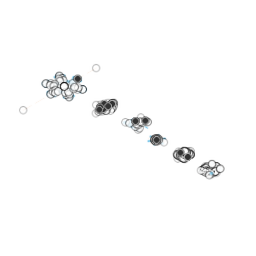
day2_sketches (Autodesk Fusion 360 design; units mm, degrees)
part number: 2026-04-13-20-48-34-590
Autodesk Fusion 360 part; units mm, degrees
(part 1 of 3)
sketch "Sketch1" plane through (0, 0, 0) normal (0, 0, 1) x (1, 0, 0)
  circle A0 centre (0, 0) radius 14
  circle A1 centre (0, 0) radius 20
  circle A2 centre (0, 0) radius 73 construction
  arc A3 (73, 0) -> (70.5126, 18.8938) centre (0, 0) ccw construction
  line L0 (0, 0) -> (73, 0) construction
  line L1 (19.3185, 5.1764) -> (34.7733, 9.3175)
  line L2 (19.3185, -5.1764) -> (34.7733, -9.3175)
  line L3 (34.7733, 9.3175) -> (73, 0)
  line L4 (34.7733, -9.3175) -> (73, 0)
  arc A4 (34.7733, -9.3175) -> (34.7733, 9.3175) centre (0, 0) ccw
  line L5 (5.1764, 19.3185) -> (9.3175, 34.7733)
  arc A5 (25.4558, 25.4558) -> (9.3175, 34.7733) centre (0, 0) ccw
  line L6 (14.1421, 14.1421) -> (25.4558, 25.4558)
  line L7 (25.4558, 25.4558) -> (36.5, 63.2199)
  line L8 (9.3175, 34.7733) -> (36.5, 63.2199)
  line L9 (-14.1421, 14.1421) -> (-25.4558, 25.4558)
  arc A6 (-9.3175, 34.7733) -> (-25.4558, 25.4558) centre (0, 0) ccw
  line L10 (-5.1764, 19.3185) -> (-9.3175, 34.7733)
  line L11 (-9.3175, 34.7733) -> (-36.5, 63.2199)
  line L12 (-25.4558, 25.4558) -> (-36.5, 63.2199)
  line L13 (-19.3185, -5.1764) -> (-34.7733, -9.3175)
  arc A7 (-34.7733, 9.3175) -> (-34.7733, -9.3175) centre (0, 0) ccw
  line L14 (-19.3185, 5.1764) -> (-34.7733, 9.3175)
  line L15 (-34.7733, 9.3175) -> (-73, 0)
  line L16 (-34.7733, -9.3175) -> (-73, 0)
  line L17 (-5.1764, -19.3185) -> (-9.3175, -34.7733)
  arc A8 (-25.4558, -25.4558) -> (-9.3175, -34.7733) centre (0, 0) ccw
  line L18 (-14.1421, -14.1421) -> (-25.4558, -25.4558)
  line L19 (-25.4558, -25.4558) -> (-36.5, -63.2199)
  line L20 (-9.3175, -34.7733) -> (-36.5, -63.2199)
  line L21 (14.1421, -14.1421) -> (25.4558, -25.4558)
  arc A9 (9.3175, -34.7733) -> (25.4558, -25.4558) centre (0, 0) ccw
  line L22 (5.1764, -19.3185) -> (9.3175, -34.7733)
  line L23 (9.3175, -34.7733) -> (36.5, -63.2199)
  line L24 (25.4558, -25.4558) -> (36.5, -63.2199)
  line L25 (300, 50) -> (350, 50) construction
  line L26 (325, 70) -> (325, 30) construction
  line L27 (300, 50) -> (300.1627, 50)
  line L28 (300.1627, 50) -> (300.1627, -30) construction
  line L29 (300.1627, -30) -> (300, -30)
  line L30 (300, -30) -> (300, 50) construction
  line L31 (260, 10) -> (370.6155, 10) construction
  arc A10 (341.6667, -42.4722) -> (308.3333, -42.4722) centre (325, -67.4166) ccw
  arc A11 (359.0765, 38.2526) -> (355.3385, 36.4191) centre (370.6155, 10) ccw
  arc A12 (300.1627, -15.0009) -> (300, -15) centre (300, -30) ccw
  arc A13 (285, -30) -> (315, -30) centre (300, -30) ccw
  arc A14 (300.1627, -20.0013) -> (300, -20) centre (300, -30) ccw
  arc A15 (290, -30) -> (310, -30) centre (300, -30) ccw
  arc A16 (340, -30) -> (360, -30) centre (350, -30) ccw
  arc A17 (335, -30) -> (365, -30) centre (350, -30) ccw
  line L32 (275, -30) -> (375, -30) construction
  arc A18 (310, -30) -> (290, -30) centre (300, -30) ccw
  arc A19 (315, -30) -> (285, -30) centre (300, -30) ccw
  arc A20 (308.3333, -17.5278) -> (341.6667, -17.5278) centre (325, 7.4166) ccw
  arc A21 (365, -30) -> (335, -30) centre (350, -30) ccw
  arc A22 (360, -30) -> (340, -30) centre (350, -30) ccw
  arc A23 (341.6667, 37.5278) -> (308.3333, 37.5278) centre (325, 12.5834) ccw
  arc A24 (308.3333, 62.4722) -> (341.6667, 62.4722) centre (325, 87.4166) ccw
  arc A25 (335, 50) -> (365, 50) centre (350, 50) ccw
  arc A26 (365, 50) -> (335, 50) centre (350, 50) ccw
  arc A27 (360, 50) -> (340, 50) centre (350, 50) ccw
  arc A28 (340, 50) -> (360, 50) centre (350, 50) ccw
  arc A29 (285, 50) -> (315, 50) centre (300, 50) ccw
  arc A30 (315, 50) -> (285, 50) centre (300, 50) ccw
  arc A31 (310, 50) -> (290, 50) centre (300, 50) ccw
  arc A32 (290, 50) -> (310, 50) centre (300, 50) ccw
  arc A33 (356.8719, 36.6667) -> (356.8719, -16.6667) centre (370.6155, 10) ccw
  arc A34 (293.1282, -16.6667) -> (293.1282, 36.6667) centre (279.3845, 10) ccw
  dimension "d7" = 360
  constraint coincident A0.centre A1.centre
  constraint concentric A1 A2
  constraint concentric A1 A4
  constraint coincident A2 A3.start
  constraint coincident A1 L2.start
  constraint coincident A1 L1.start
  constraint horizontal L25
  constraint perpendicular L25 L26
  constraint horizontal L27
  constraint vertical L28
  constraint horizontal L29
  constraint vertical L30
  constraint perpendicular L28 L31
  constraint coincident L31.end A11.centre
  constraint tangent A10 A17
  constraint tangent A10 A13
  constraint coincident A10.end A13
  constraint coincident A10.start A17
  constraint coincident L28 A12.start
  constraint coincident L30 A12.end
  constraint concentric A12 A13
  constraint coincident L28 A14.start
  constraint coincident L30 A14.end
  constraint concentric A14 A15
  constraint perpendicular L28 L32
  constraint symmetric A10.end L32 A20.start
  constraint symmetric A10.start L32 A20.end
  constraint symmetric A10 L32 A20
  constraint symmetric A13.end L32 A19.start
  constraint symmetric A17.start L32 A21.end
  constraint symmetric A13.start L32 A19.end
  constraint symmetric A13 L32 A19
  constraint symmetric A15.end L32 A18.start
  constraint symmetric A15.start L32 A18.end
  constraint symmetric A15 L32 A18
  constraint symmetric A16.end L32 A22.start
  constraint symmetric A16.start L32 A22.end
  constraint symmetric A16 L32 A22
  constraint symmetric A17.end L32 A21.start
  constraint symmetric A17 L32 A21
  constraint symmetric L31 A10.end A24.start
  constraint symmetric L31 A10.start A24.end
  constraint symmetric L31 A10 A24
  constraint symmetric L31 A13.end A29.end
  constraint symmetric L31 A17.start A25.start
  constraint symmetric L31 A13.start A29.start
  constraint symmetric L31 A13 A30
  constraint symmetric L31 A15.end A31.start
  constraint symmetric L31 A15.start A31.end
  constraint symmetric L31 A15 A31
  constraint symmetric L31 A16.end A27.start
  constraint symmetric L31 A16.start A27.end
  constraint symmetric L31 A16 A27
  constraint symmetric L31 A17.end A25.end
  constraint symmetric L31 A17 A26
  constraint symmetric L31 A18 A32
  constraint symmetric L31 A19 A29
  constraint symmetric L31 A20.end A23.start
  constraint symmetric L31 A20.start A23.end
  constraint symmetric L31 A20 A23
  constraint symmetric L31 A21 A25
  constraint symmetric L31 A22 A28
  constraint tangent A25 A33
  constraint coincident A21 A33.end
  constraint coincident A25 A33.start
  constraint coincident L31 A34.centre
  constraint tangent A29 A34
  constraint coincident A29 A34.end
  constraint coincident A19 A34.start
sketch "Sketch2" plane through (0, 0, 0) normal (0, 0, 1) x (1, 0, 0)
  line L0 (-379.9986, -15) -> (-214.9986, -15)
  line L1 (-214.9986, -15) -> (-214.9986, -5.344)
  line L2 (-219.9986, -0.344) -> (-226.0015, -0.344)
  line L3 (-379.9986, -5.344) -> (-379.9986, -15)
  arc A0 (-214.9986, -5.344) -> (-219.9986, -0.344) centre (-219.9986, -5.344) ccw
  arc A1 (-374.9986, -0.344) -> (-379.9986, -5.344) centre (-374.9986, -5.344) ccw
  circle A2 centre (-326, 69) radius 16
  circle A3 centre (-326, 69) radius 35
  line L4 (-326, 69) -> (-325.9604, 133.975) construction
  line L5 (-325.9604, 133.975) -> (-271.0015, 133.9415) construction
  circle A4 centre (-271.0015, 133.9415) radius 12
  circle A5 centre (-271.0015, 133.9415) radius 25
  line L6 (-246.0015, 133.9415) -> (-246.0015, 132)
  line L7 (-271.0015, 133.9415) -> (-241, 133.9415) construction
  line L8 (-246.0015, 133.9415) -> (-246.0015, 19.656)
  arc A6 (-246.0015, 19.656) -> (-226.0015, -0.344) centre (-226.0015, 19.656) ccw
  arc A7 (-328.4008, 103.9176) -> (-295.9182, 135.9805) centre (-330.8016, 138.8351) ccw
  line L9 (-261.0635, 111.0016) -> (-261.0635, 92.814)
  line L10 (-326, 69) -> (-180, 68.9111) construction
  line L11 (-180, 68.9111) -> (-206.1133, 68.927)
  line L12 (-290.1965, 84.814) -> (-269.0635, 84.814)
  line L13 (-290.2427, 53.1529) -> (-269.8408, 53.2148)
  line L14 (-261.777, 8.7586) -> (-261.8166, 45.2235)
  line L15 (-374.9986, -0.344) -> (-225, -0.344)
  arc A8 (-360.0045, 60.712) -> (-268.3878, 0.8714) centre (-282.2799, 79.656) ccw
  arc A9 (-268.3878, 0.8714) -> (-261.777, 8.7586) centre (-269.777, 8.7499) ccw
  arc A10 (-261.8166, 45.2235) -> (-269.8408, 53.2148) centre (-269.8166, 45.2148) ccw
  arc A11 (-269.0635, 84.814) -> (-261.0635, 92.814) centre (-269.0635, 92.814) ccw
  arc A12 (-290.2427, 53.1529) -> (-296.8755, 49.5896) centre (-290.2184, 45.153) ccw
  arc A13 (-296.8576, 88.3835) -> (-290.1965, 84.814) centre (-290.1965, 92.814) ccw
  arc A14 (-338.8484, -0.344) -> (-332.563, 17.4338) centre (-338.8484, 9.656) ccw
  line L16 (-650, 60) -> (-698, 60)
  circle A15 centre (-698, 60) radius 7.5
  line L17 (-650, 60) -> (-650, 108) construction
  line L18 (-664, 108) -> (-664, 94)
  line L19 (-698, 74) -> (-684, 74)
  arc A16 (-684, 74) -> (-664, 94) centre (-684, 94) ccw
  arc A17 (-697.4782, 13.3614) -> (-703.1993, 47.0013) centre (-710.6269, 28.4316) ccw
  arc A18 (-703.9799, -1.4739) -> (-650, -54) centre (-650, 0) ccw
  arc A19 (-698, 74) -> (-703.1993, 47.0013) centre (-698, 60) ccw
  arc A20 (-650, 122) -> (-664, 108) centre (-650, 108) ccw
  arc A21 (-650, 115.5) -> (-650, 100.5) centre (-650, 108) ccw
  line L20 (-650, 130) -> (-650, -90) construction
  line L21 (-650, 0) -> (-736.423, 0) construction
  line L22 (-650, 0) -> (-677, -46.7654) construction
  arc A22 (-676, 0) -> (-663, -22.5167) centre (-650, 0) ccw
  arc A23 (-694, 0) -> (-672, -38.1051) centre (-650, 0) ccw
  arc A24 (-676, 0) -> (-694, 0) centre (-685, 0) ccw
  arc A25 (-672, -38.1051) -> (-663, -22.5167) centre (-667.5, -30.3109) ccw
  line L23 (-660, 60) -> (-660, 20)
  arc A26 (-662, 16) -> (-660, 20) centre (-665, 20) ccw
  arc A27 (-650, 70) -> (-650, 50) centre (-650, 60) ccw
  arc A28 (-662, 16) -> (-650, -20) centre (-650, 0) ccw
  arc A29 (-650, 35) -> (-650, -35) centre (-650, 0) ccw construction
  arc A30 (-650, 100.5) -> (-650, 115.5) centre (-650, 108) ccw
  line L24 (-636, 108) -> (-636, 94)
  arc A31 (-636, 108) -> (-650, 122) centre (-650, 108) ccw
  arc A32 (-636, 94) -> (-616, 74) centre (-616, 94) ccw
  line L25 (-602, 74) -> (-616, 74)
  arc A33 (-596.8007, 47.0013) -> (-602, 74) centre (-602, 60) ccw
  circle A34 centre (-602, 60) radius 7.5
  arc A35 (-650, 50) -> (-650, 70) centre (-650, 60) ccw
  line L26 (-640, 60) -> (-640, 20)
  arc A36 (-596.8007, 47.0013) -> (-602.5218, 13.3614) centre (-589.3731, 28.4316) ccw
  arc A37 (-650, -54) -> (-596.0201, -1.4739) centre (-650, 0) ccw
  arc A38 (-628, -38.1051) -> (-606, 0) centre (-650, 0) ccw
  arc A39 (-637, -22.5167) -> (-624, 0) centre (-650, 0) ccw
  arc A40 (-637, -22.5167) -> (-628, -38.1051) centre (-632.5, -30.3109) ccw
  arc A41 (-606, 0) -> (-624, 0) centre (-615, 0) ccw
  arc A42 (-650, -20) -> (-638, 16) centre (-650, 0) ccw
  arc A43 (-640, 20) -> (-638, 16) centre (-635, 20) ccw
  arc A44 (-596.0201, -1.4739) -> (-602.5218, 13.3614) centre (-615.013, -0.9553) ccw
  arc A45 (-697.4782, 13.3614) -> (-703.9799, -1.4739) centre (-684.987, -0.9553) ccw
  circle A46 centre (-1125, 0) radius 75
  circle A47 centre (-1125, 0) radius 90
  line L27 (-1124.6288, 388.2293) -> (-1124.6288, -500) construction
  line L28 (-1139.6288, 121.5732) -> (-1139.6288, 88.8031)
  line L29 (-1109.6288, 121.5732) -> (-1109.6288, 88.8031)
  circle A48 centre (-1124.6288, 163.9996) radius 30
  arc A49 (-1169.2171, 157.9267) -> (-1080.0684, 157.7249) centre (-1124.6288, 163.9996) ccw
  arc A50 (-1080.0684, 157.7249) -> (-1169.2171, 157.9267) centre (-1125, 0) ccw
  circle A51 centre (-1266.8422, 82.3213) radius 30
  arc A52 (-1239.128, 117.7744) -> (-1283.8771, 40.6702) centre (-1125, 0) ccw
  arc A53 (-1283.8771, 40.6702) -> (-1239.128, 117.7744) centre (-1266.8422, 82.3213) ccw
  line L30 (-1222.5998, 74.0985) -> (-1194.2202, 57.7134)
  line L31 (-1237.5998, 48.1177) -> (-1209.2202, 31.7327)
  circle A54 centre (-1267.2134, -81.6783) radius 30
  arc A55 (-1284.0596, -39.9505) -> (-1239.66, -117.2565) centre (-1125, 0) ccw
  arc A56 (-1239.66, -117.2565) -> (-1284.0596, -39.9505) centre (-1267.2134, -81.6783) ccw
  line L32 (-1237.9711, -47.4747) -> (-1209.5914, -31.0897)
  line L33 (-1222.9711, -73.4555) -> (-1194.5914, -57.0705)
  circle A57 centre (-1125.3712, -163.9996) radius 30
  arc A58 (-1169.9316, -157.7249) -> (-1080.7829, -157.9267) centre (-1125, 0) ccw
  arc A59 (-1080.7829, -157.9267) -> (-1169.9316, -157.7249) centre (-1125.3712, -163.9996) ccw
  line L34 (-1140.3712, -121.5732) -> (-1140.3712, -88.8031)
  line L35 (-1110.3712, -121.5732) -> (-1110.3712, -88.8031)
  circle A60 centre (-983.1578, -82.3213) radius 30
  arc A61 (-1010.872, -117.7744) -> (-966.1229, -40.6702) centre (-1125, 0) ccw
  arc A62 (-966.1229, -40.6702) -> (-1010.872, -117.7744) centre (-983.1578, -82.3213) ccw
  line L36 (-1027.4002, -74.0985) -> (-1055.7798, -57.7134)
  line L37 (-1012.4002, -48.1177) -> (-1040.7798, -31.7327)
  circle A63 centre (-982.7866, 81.6783) radius 30
  arc A64 (-965.9404, 39.9505) -> (-1010.34, 117.2565) centre (-1125, 0) ccw
  arc A65 (-1010.34, 117.2565) -> (-965.9404, 39.9505) centre (-982.7866, 81.6783) ccw
  line L38 (-1012.0289, 47.4747) -> (-1040.4086, 31.0897)
  line L39 (-1027.0289, 73.4555) -> (-1055.4086, 57.0705)
  line L40 (597.5, -18) -> (608.5, -18)
  line L41 (609, -17.5) -> (609, -14.5)
  line L42 (608.5, -14) -> (597.5, -14)
  line L43 (597, -14.5) -> (597, -17.5)
  line L44 (597.5, -13) -> (604.5, -13)
  line L45 (605, -12.5) -> (605, -9.5)
  line L46 (604.5, -9) -> (597.5, -9)
  line L47 (597, -9.5) -> (597, -12.5)
  line L48 (597.5, -8) -> (602.5, -8)
  line L49 (603, -7.5) -> (603, -4.5)
  line L50 (602.5, -4) -> (597.5, -4)
  line L51 (597, -4.5) -> (597, -7.5)
  line L52 (604.5, -4) -> (607.5, -4)
  line L53 (608, -4.5) -> (608, -7.5)
  line L54 (607.5, -8) -> (604.5, -8)
  line L55 (604, -7.5) -> (604, -4.5)
  line L56 (612.5, -8) -> (609.5, -8)
  line L57 (609, -7.5) -> (609, -4.5)
  line L58 (613, -4.5) -> (613, -7.5)
  line L59 (609.5, -4) -> (612.5, -4)
  line L60 (617.5, -8) -> (614.5, -8)
  line L61 (614, -7.5) -> (614, -4.5)
  line L62 (618, -4.5) -> (618, -7.5)
  line L63 (614.5, -4) -> (617.5, -4)
  line L64 (622.5, -8) -> (619.5, -8)
  line L65 (619, -7.5) -> (619, -4.5)
  line L66 (623, -4.5) -> (623, -7.5)
  line L67 (619.5, -4) -> (622.5, -4)
  line L68 (627.5, -8) -> (624.5, -8)
  line L69 (624, -7.5) -> (624, -4.5)
  line L70 (628, -4.5) -> (628, -7.5)
  line L71 (624.5, -4) -> (627.5, -4)
  line L72 (632.5, -8) -> (629.5, -8)
  line L73 (629, -7.5) -> (629, -4.5)
  line L74 (633, -4.5) -> (633, -7.5)
  line L75 (629.5, -4) -> (632.5, -4)
  line L76 (637.5, -8) -> (634.5, -8)
  line L77 (634, -7.5) -> (634, -4.5)
  line L78 (638, -4.5) -> (638, -7.5)
  line L79 (634.5, -4) -> (637.5, -4)
  line L80 (642.5, -8) -> (639.5, -8)
  line L81 (639, -7.5) -> (639, -4.5)
  line L82 (643, -4.5) -> (643, -7.5)
  line L83 (639.5, -4) -> (642.5, -4)
  line L84 (647.5, -8) -> (644.5, -8)
  line L85 (644, -7.5) -> (644, -4.5)
  line L86 (648, -4.5) -> (648, -7.5)
  line L87 (644.5, -4) -> (647.5, -4)
  line L88 (652.5, -8) -> (649.5, -8)
  line L89 (649, -7.5) -> (649, -4.5)
  line L90 (653, -4.5) -> (653, -7.5)
  line L91 (649.5, -4) -> (652.5, -4)
  line L92 (657.5, -8) -> (654.5, -8)
  line L93 (654, -7.5) -> (654, -4.5)
  line L94 (658, -4.5) -> (658, -7.5)
  line L95 (654.5, -4) -> (657.5, -4)
  line L96 (662.5, -8) -> (659.5, -8)
  line L97 (659, -7.5) -> (659, -4.5)
  line L98 (663, -4.5) -> (663, -7.5)
  line L99 (659.5, -4) -> (662.5, -4)
  line L100 (667.5, -8) -> (664.5, -8)
  line L101 (664, -7.5) -> (664, -4.5)
  line L102 (668, -4.5) -> (668, -7.5)
  line L103 (664.5, -4) -> (667.5, -4)
  line L104 (606.5, -9) -> (609.5, -9)
  line L105 (610, -9.5) -> (610, -12.5)
  line L106 (609.5, -13) -> (606.5, -13)
  line L107 (606, -12.5) -> (606, -9.5)
  line L108 (614.5, -13) -> (611.5, -13)
  line L109 (611, -12.5) -> (611, -9.5)
  line L110 (611.5, -9) -> (614.5, -9)
  line L111 (615, -9.5) -> (615, -12.5)
  line L112 (619.5, -13) -> (616.5, -13)
  line L113 (616, -12.5) -> (616, -9.5)
  line L114 (616.5, -9) -> (619.5, -9)
  line L115 (620, -9.5) -> (620, -12.5)
  line L116 (624.5, -13) -> (621.5, -13)
  line L117 (621, -12.5) -> (621, -9.5)
  line L118 (621.5, -9) -> (625, -9)
  line L119 (625, -9) -> (625, -12.5)
  line L120 (629.5, -13) -> (626.5, -13)
  line L121 (626, -12.5) -> (626, -9.5)
  line L122 (626.5, -9) -> (629.5, -9)
  line L123 (630, -9.5) -> (630, -12.5)
  line L124 (634.5, -13) -> (631.5, -13)
  line L125 (631, -12.5) -> (631, -9.5)
  line L126 (631.5, -9) -> (634.5, -9)
  line L127 (635, -9.5) -> (635, -12.5)
  line L128 (639.5, -13) -> (636.5, -13)
  line L129 (636, -12.5) -> (636, -9.5)
  line L130 (636.5, -9) -> (639.5, -9)
  line L131 (640, -9.5) -> (640, -12.5)
  line L132 (644.5, -13) -> (641.5, -13)
  line L133 (641, -12.5) -> (641, -9.5)
  line L134 (641.5, -9) -> (644.5, -9)
  line L135 (645, -9.5) -> (645, -12.5)
  line L136 (649.5, -13) -> (646.5, -13)
  line L137 (646, -12.5) -> (646, -9.5)
  line L138 (646.5, -9) -> (649.5, -9)
  line L139 (650, -9.5) -> (650, -12.5)
  line L140 (654.5, -13) -> (651.5, -13)
  line L141 (651, -12.5) -> (651, -9.5)
  line L142 (651.5, -9) -> (654.5, -9)
  line L143 (655, -9.5) -> (655, -12.5)
  line L144 (659.5, -13) -> (656.5, -13)
  line L145 (656, -12.5) -> (656, -9.5)
  line L146 (656.5, -9) -> (659.5, -9)
  line L147 (660, -9.5) -> (660, -12.5)
  line L148 (661.5, -9) -> (667.5, -9)
  line L149 (668, -9.5) -> (668, -12.5)
  line L150 (667.5, -13) -> (661.5, -13)
  line L151 (661, -12.5) -> (661, -9.5)
  line L152 (610.5, -14) -> (613.5, -14)
  line L153 (614, -14.5) -> (614, -17.5)
  line L154 (613.5, -18) -> (610.5, -18)
  line L155 (610, -17.5) -> (610, -14.5)
  line L156 (618.5, -18) -> (615.5, -18)
  line L157 (615, -17.5) -> (615, -14.5)
  line L158 (615.5, -14) -> (618.5, -14)
  line L159 (619, -14.5) -> (619, -17.5)
  line L160 (623.5, -18) -> (620.5, -18)
  line L161 (620, -17.5) -> (620, -14.5)
  line L162 (620.5, -14) -> (623.5, -14)
  line L163 (624, -14.5) -> (624, -17.5)
  line L164 (628.5, -18) -> (625.5, -18)
  line L165 (625, -17.5) -> (625, -14.5)
  line L166 (625.5, -14) -> (628.5, -14)
  line L167 (629, -14.5) -> (629, -17.5)
  line L168 (633.5, -18) -> (630.5, -18)
  line L169 (630, -17.5) -> (630, -14)
  line L170 (630, -14) -> (633.5, -14)
  line L171 (634, -14.5) -> (634, -17.5)
  line L172 (638.5, -18) -> (635.5, -18)
  line L173 (635, -17.5) -> (635, -14.5)
  line L174 (635.5, -14) -> (638.5, -14)
  line L175 (639, -14.5) -> (639, -17.5)
  line L176 (643.5, -18) -> (640.5, -18)
  line L177 (640, -17.5) -> (640, -14.5)
  line L178 (640.5, -14) -> (643.5, -14)
  line L179 (644, -14.5) -> (644, -17.5)
  line L180 (648.5, -18) -> (645.5, -18)
  line L181 (645, -17.5) -> (645, -14.5)
  line L182 (645.5, -14) -> (648.5, -14)
  line L183 (649, -14.5) -> (649, -17.5)
  line L184 (653.5, -18) -> (650.5, -18)
  line L185 (650, -17.5) -> (650, -14.5)
  line L186 (650.5, -14) -> (653.5, -14)
  line L187 (654, -14.5) -> (654, -17.5)
  line L188 (658.5, -18) -> (655.5, -18)
  line L189 (655, -17.5) -> (655, -14.5)
  line L190 (655.5, -14) -> (658.5, -14)
  line L191 (659, -14.5) -> (659, -17.5)
  line L192 (660.5, -14) -> (667.5, -14)
  line L193 (668, -14.5) -> (668, -17.5)
  line L194 (667.5, -18) -> (660.5, -18)
  line L195 (660, -17.5) -> (660, -14.5)
  line L196 (597.5, -3) -> (599.5, -3)
  line L197 (600, -2.5) -> (600, 0.5)
  line L198 (599.5, 1) -> (597.5, 1)
  line L199 (597, 0.5) -> (597, -2.5)
  line L200 (601.5, 1) -> (604.5, 1)
  line L201 (605, 0.5) -> (605, -2.5)
  line L202 (604.5, -3) -> (601.5, -3)
  line L203 (601, -2.5) -> (601, 0.5)
  line L204 (609.5, -3) -> (606.5, -3)
  line L205 (606, -2.5) -> (606, 0.5)
  line L206 (606.5, 1) -> (609.5, 1)
  line L207 (610, 0.5) -> (610, -2.5)
  line L208 (614.5, -3) -> (611.5, -3)
  line L209 (611, -2.5) -> (611, 0.5)
  line L210 (611.5, 1) -> (614.5, 1)
  line L211 (615, 0.5) -> (615, -2.5)
  line L212 (619.5, -3) -> (616.5, -3)
  line L213 (616, -2.5) -> (616, 0.5)
  line L214 (616.5, 1) -> (619.5, 1)
  line L215 (620, 0.5) -> (620, -2.5)
  line L216 (624.5, -3) -> (621.5, -3)
  line L217 (621, -2.5) -> (621, 0.5)
  line L218 (621.5, 1) -> (624.5, 1)
  line L219 (625, 0.5) -> (625, -2.5)
  line L220 (629.5, -3) -> (626.5, -3)
  line L221 (626, -2.5) -> (626, 0.5)
  line L222 (626.5, 1) -> (629.5, 1)
  line L223 (630, 0.5) -> (630, -2.5)
  line L224 (634.5, -3) -> (631.5, -3)
  line L225 (631, -2.5) -> (631, 0.5)
  line L226 (631.5, 1) -> (634.5, 1)
  line L227 (635, 0.5) -> (635, -2.5)
  line L228 (639.5, -3) -> (636.5, -3)
  line L229 (636, -2.5) -> (636, 0.5)
  line L230 (636.5, 1) -> (639.5, 1)
  line L231 (640, 0.5) -> (640, -2.5)
  line L232 (644.5, -3) -> (641.5, -3)
  line L233 (641, -2.5) -> (641, 0.5)
  line L234 (641.5, 1) -> (644.5, 1)
  line L235 (645, 0.5) -> (645, -2.5)
  line L236 (649.5, -3) -> (646.5, -3)
  line L237 (646, -2.5) -> (646, 0.5)
  line L238 (646.5, 1) -> (649.5, 1)
  line L239 (650, 0.5) -> (650, -2.5)
  line L240 (654.5, -3) -> (651.5, -3)
  line L241 (651, -2.5) -> (651, 0.5)
  line L242 (651.5, 1) -> (654.5, 1)
  line L243 (655, 0.5) -> (655, -2.5)
  line L244 (659.5, -3) -> (656.5, -3)
  line L245 (656, -2.5) -> (656, 0.5)
  line L246 (656.5, 1) -> (659.5, 1)
  line L247 (660, 0.5) -> (660, -2.5)
  line L248 (661.5, -3) -> (667.5, -3)
  line L249 (668, -2.5) -> (668, 0.5)
  line L250 (667.5, 1) -> (661.5, 1)
  line L251 (661, 0.5) -> (661, -2.5)
  line L252 (599.5007, 2) -> (602.5007, 2)
  line L253 (603.0007, 2.5) -> (603.0007, 4.5)
  line L254 (602.5007, 5) -> (599.5007, 5)
  line L255 (599.0007, 4.5) -> (599.0007, 2.5)
  line L256 (604.5007, 2) -> (607.5007, 2)
  line L257 (608.0007, 2.5) -> (608.0007, 4.5)
  line L258 (604.0007, 4.5) -> (604.0007, 2.5)
  line L259 (607.5007, 5) -> (604.5007, 5)
  line L260 (609.5007, 2) -> (612.5007, 2)
  line L261 (613.0007, 2.5) -> (613.0007, 4.5)
  line L262 (609.0007, 4.5) -> (609.0007, 2.5)
  line L263 (612.5007, 5) -> (609.5007, 5)
  line L264 (614.5007, 2) -> (617.5007, 2)
  line L265 (618.0007, 2.5) -> (618.0007, 4.5)
  line L266 (614.0007, 4.5) -> (614.0007, 2.5)
  line L267 (617.5007, 5) -> (614.5007, 5)
  line L268 (619.5007, 2) -> (622.5007, 2)
  line L269 (623.0007, 2.5) -> (623.0007, 4.5)
  line L270 (619.0007, 4.5) -> (619.0007, 2.5)
  line L271 (622.5007, 5) -> (619.5007, 5)
  line L272 (624.5007, 2) -> (627.5007, 2)
  line L273 (628.0007, 2.5) -> (628.0007, 4.5)
  line L274 (624.0007, 4.5) -> (624.0007, 2.5)
  line L275 (627.5007, 5) -> (624.5007, 5)
  line L276 (629.5007, 2) -> (632.5007, 2)
  line L277 (633.0007, 2.5) -> (633.0007, 4.5)
  line L278 (629.0007, 4.5) -> (629.0007, 2.5)
  line L279 (632.5007, 5) -> (629.5007, 5)
  line L280 (634.5007, 2) -> (637.5007, 2)
  line L281 (638.0007, 2.5) -> (638.0007, 4.5)
  line L282 (634.0007, 4.5) -> (634.0007, 2.5)
  line L283 (637.5007, 5) -> (634.5007, 5)
  line L284 (639.5007, 2) -> (642.5007, 2)
  line L285 (643.0007, 2.5) -> (643.0007, 4.5)
  line L286 (639.0007, 4.5) -> (639.0007, 2.5)
  line L287 (642.5007, 5) -> (639.5007, 5)
  line L288 (644.5007, 2) -> (647.5007, 2)
  line L289 (648.0007, 2.5) -> (648.0007, 4.5)
  line L290 (644.0007, 4.5) -> (644.0007, 2.5)
  line L291 (647.5007, 5) -> (644.5007, 5)
  line L292 (649.5007, 2) -> (652.5007, 2)
  line L293 (653.0007, 2.5) -> (653.0007, 4.5)
  line L294 (649.0007, 4.5) -> (649.0007, 2.5)
  line L295 (652.5007, 5) -> (649.5007, 5)
  line L296 (654.5007, 2) -> (657.5007, 2)
  line L297 (658.0007, 2.5) -> (658.0007, 4.5)
  line L298 (654.0007, 4.5) -> (654.0007, 2.5)
  line L299 (657.5007, 5) -> (654.5007, 5)
  line L300 (659.5007, 2) -> (662.5007, 2)
  line L301 (663.0007, 2.5) -> (663.0007, 4.5)
  line L302 (659.0007, 4.5) -> (659.0007, 2.5)
  line L303 (662.5007, 5) -> (659.5007, 5)
  line L304 (664.5007, 2) -> (667.5007, 2)
  line L305 (668.0007, 2.5) -> (668.0007, 4.5)
  line L306 (664.0007, 4.5) -> (664.0007, 2.5)
  line L307 (667.5007, 5) -> (664.5007, 5)
  line L308 (669.5007, 2) -> (672.5007, 2)
  line L309 (673.0007, 2.5) -> (673.0007, 4.5)
  line L310 (669.0007, 4.5) -> (669.0007, 2.5)
  line L311 (672.5007, 5) -> (669.5007, 5)
  line L312 (674.5007, 2) -> (677.5007, 2)
  line L313 (678.0007, 2.5) -> (678.0007, 4.5)
  line L314 (674.0007, 4.5) -> (674.0007, 2.5)
  line L315 (677.5007, 5) -> (674.5007, 5)
  line L316 (679.5007, 2) -> (682.5007, 2)
  line L317 (683.0007, 2.5) -> (683.0007, 4.5)
  line L318 (679.0007, 4.5) -> (679.0007, 2.5)
  line L319 (682.5007, 5) -> (679.5007, 5)
  line L320 (684.5007, 2) -> (687.5007, 2)
  line L321 (688.0007, 2.5) -> (688.0007, 4.5)
  line L322 (684.0007, 4.5) -> (684.0007, 2.5)
  line L323 (687.5007, 5) -> (684.5007, 5)
  line L324 (669.5, 1) -> (672.5, 1)
  line L325 (673, 0.5) -> (673, -2.5)
  line L326 (672.5, -3) -> (669.5, -3)
  line L327 (669, -2.5) -> (669, 0.5)
  line L328 (674.5, 1) -> (677.5, 1)
  line L329 (678, 0.5) -> (678, -2.5)
  line L330 (677.5, -3) -> (674.5, -3)
  line L331 (674, -2.5) -> (674, 0.5)
  line L332 (679.5, 1) -> (682.5, 1)
  line L333 (683, 0.5) -> (683, -2.5)
  line L334 (682.5, -3) -> (679.5, -3)
  line L335 (679, -2.5) -> (679, 0.5)
  line L336 (684.5, 1) -> (687.5, 1)
  line L337 (688, 0.5) -> (688, -2.5)
  line L338 (687.5, -3) -> (684.5, -3)
  line L339 (684, -2.5) -> (684, 0.5)
  line L340 (669.5, -4) -> (672.5, -4)
  line L341 (673, -4.5) -> (673, -7.5)
  line L342 (672.5, -8) -> (669.5, -8)
  line L343 (669, -7.5) -> (669, -4.5)
  line L344 (677.5, -8) -> (674.5, -8)
  line L345 (674, -7.5) -> (674, -4.5)
  line L346 (678, -4.5) -> (678, -7.5)
  line L347 (674.5, -4) -> (677.5, -4)
  line L348 (682.5, -8) -> (679.5, -8)
  line L349 (679, -7.5) -> (679, -4.5)
  line L350 (683, -4.5) -> (683, -7.5)
  line L351 (679.5, -4) -> (682.5, -4)
  line L352 (684.5, -4) -> (687.5, -4)
  line L353 (672.5, -13) -> (669.5, -13)
  line L354 (669, -12.5) -> (669, -9.5)
  line L355 (673, -9.5) -> (673, -12.5)
  line L356 (669.5, -9) -> (672.5, -9)
  line L357 (677.5, -13) -> (674.5, -13)
  line L358 (674, -12.5) -> (674, -9.5)
  line L359 (678, -9.5) -> (678, -12.5)
  line L360 (674.5, -9) -> (677.5, -9)
  line L361 (683, -13) -> (679.5, -13)
  line L362 (679, -12.5) -> (679, -9.5)
  line L363 (683, -9.5) -> (683, -13)
  line L364 (679.5, -9) -> (682.5, -9)
  line L365 (687.5, -13) -> (684.5, -13)
  line L366 (684, -12.5) -> (684, -4.5)
  line L367 (688, -4.5) -> (688, -12.5)
  line L368 (672.5, -18) -> (669.5, -18)
  line L369 (669, -17.5) -> (669, -14.5)
  line L370 (673, -14.5) -> (673, -17.5)
  line L371 (669.5, -14) -> (672.5, -14)
  line L372 (677.5, -18) -> (674.5, -18)
  line L373 (674, -17.5) -> (674, -14.5)
  line L374 (678, -14.5) -> (678, -17.5)
  line L375 (674.5, -14) -> (677.5, -14)
  line L376 (682.5, -18) -> (679.5, -18)
  line L377 (679, -17.5) -> (679, -14.5)
  line L378 (683, -14.5) -> (683, -17.5)
  line L379 (679.5, -14) -> (682.5, -14)
  line L380 (677.5, -23) -> (669.5, -23)
  line L381 (669, -22.5) -> (669, -19.5)
  line L382 (678, -19.5) -> (678, -22.5)
  line L383 (669.5, -19) -> (677.5, -19)
  line L384 (682.5, -23) -> (679.5, -23)
  line L385 (679, -22.5) -> (679, -19.5)
  line L386 (683, -19.5) -> (683, -22.5)
  line L387 (679.5, -19) -> (682.5, -19)
  line L388 (684.5, -14) -> (687.5, -14)
  line L389 (688, -14.5) -> (688, -22.5)
  line L390 (687.5, -23) -> (684.5, -23)
  line L391 (684, -22.5) -> (684, -14.5)
  line L392 (597.5, -19) -> (600.5, -19)
  line L393 (601, -19.5) -> (601, -22.5)
  line L394 (600.5, -23) -> (597.5, -23)
  line L395 (597, -22.5) -> (597, -19.5)
  line L396 (602.5, -19) -> (605.5, -19)
  line L397 (606, -19.5) -> (606, -22.5)
  line L398 (605.5, -23) -> (602.5, -23)
  line L399 (602, -22.5) -> (602, -19.5)
  line L400 (607.5, -19) -> (610.5, -19)
  line L401 (611, -19.5) -> (611, -22.5)
  line L402 (610.5, -23) -> (607.5, -23)
  line L403 (607, -22.5) -> (607, -19.5)
  line L404 (612.5, -19) -> (615.5, -19)
  line L405 (616, -19.5) -> (616, -22.5)
  line L406 (615.5, -23) -> (612.5, -23)
  line L407 (612, -22.5) -> (612, -19.5)
  line L408 (667.5, -19) -> (664.5, -19)
  line L409 (664, -19.5) -> (664, -22.5)
  line L410 (664.5, -23) -> (667.5, -23)
  line L411 (668, -22.5) -> (668, -19.5)
  line L412 (662.5, -19) -> (659.5138, -19)
  line L413 (659.0138, -19.5) -> (659.0138, -20.202)
  line L414 (659.5138, -20.702) -> (662.5, -20.702)
  line L415 (663, -20.202) -> (663, -19.5)
  line L416 (659.5138, -21.1515) -> (662.5, -21.1515)
  line L417 (663, -21.6515) -> (663, -22.5)
  line L418 (662.5, -23) -> (659.5138, -23)
  line L419 (659.0138, -22.5) -> (659.0138, -21.6515)
  line L420 (657.5, -19) -> (654.5, -19)
  line L421 (654, -19.5) -> (654, -22.5)
  line L422 (654.5, -23) -> (657.5, -23)
  line L423 (658, -22.5) -> (658, -19.5)
  line L424 (652.5, -19) -> (649.5, -19)
  line L425 (649, -19.5) -> (649, -22.5)
  line L426 (649.5, -23) -> (652.5, -23)
  line L427 (653, -22.5) -> (653, -19.5)
  line L428 (647.5, -19) -> (644.5, -19)
  line L429 (644, -19.5) -> (644, -22.5)
  line L430 (644.5, -23) -> (647.5, -23)
  line L431 (648, -22.5) -> (648, -19.5)
  line L432 (617.5, -19) -> (642.5, -19)
  line L433 (643, -19.5) -> (643, -22.5)
  line L434 (642.5, -23) -> (617.5, -23)
  line L435 (617, -22.5) -> (617, -19.5)
  line L436 (616.5, -25) -> (641, -25)
  line L437 (643, -27) -> (643, -45)
  line L438 (641, -47) -> (617, -47)
  line L439 (615, -45) -> (615, -26.5)
  line L440 (592, 10) -> (693, 10)
  line L441 (695, 8) -> (695, -53)
  line L442 (693, -55) -> (592, -55)
  line L443 (590, -53) -> (590, 8)
  line L444 (580, 15) -> (712.1237, 15) construction
  line L445 (693, 85) -> (592, 85)
  line L446 (590, 83) -> (590, 22)
  line L447 (695, 22) -> (695, 83)
  line L448 (592, 20) -> (693, 20)
  line L449 (594, 82) -> (691, 82)
  line L450 (693, 80) -> (693, 26)
  line L451 (691, 24) -> (594, 24)
  line L452 (592, 26) -> (592, 80)
  circle A66 centre (640.4399, 83.4266) radius 1.0913
  circle A67 centre (643.5479, 83.4266) radius 0.379
  circle A68 centre (645.4808, 83.4266) radius 0.379
  line L453 (600, 2.5387) -> (602.3984, 2.5387) construction
  line L454 (602.3984, 2.5387) -> (602.3984, 4) construction
  line L455 (602.3984, 4) -> (600, 4) construction
  line L456 (600, 4) -> (600, 2.5387) construction
  line L457 (605.1445, 2.6511) -> (607.8339, 2.6511) construction
  line L458 (607.8339, 2.6511) -> (607.8339, 4.0538) construction
  line L459 (607.8339, 4.0538) -> (605.1445, 4.0538) construction
  line L460 (605.1445, 4.0538) -> (605.1445, 2.6511) construction
  line L461 (610.1729, 2.7128) -> (612.2746, 2.7122) construction
  line L462 (612.2746, 2.7122) -> (612.275, 4.1069) construction
  line L463 (612.275, 4.1069) -> (610.1732, 4.1075) construction
  line L464 (610.1732, 4.1075) -> (610.1729, 2.7128) construction
  line L465 (615, 3) -> (617, 3) construction
  line L466 (617, 3) -> (617, 4) construction
  line L467 (617, 4) -> (615, 4) construction
  line L468 (615, 4) -> (615, 3) construction
  line L469 (620, 3) -> (622, 3) construction
  line L470 (622, 3) -> (622, 4) construction
  line L471 (622, 4) -> (620, 4) construction
  line L472 (620, 4) -> (620, 3) construction
  line L473 (624.8021, 2.7475) -> (627.2182, 2.7475) construction
  line L474 (627.2182, 2.7475) -> (627.2182, 4.2315) construction
  line L475 (627.2182, 4.2315) -> (624.8021, 4.2315) construction
  line L476 (624.8021, 4.2315) -> (624.8021, 2.7475) construction
  line L477 (629.7295, 2.6714) -> (632.3739, 2.6714) construction
  line L478 (632.3739, 2.6714) -> (632.3739, 4.2315) construction
  line L479 (632.3739, 4.2315) -> (629.7295, 4.2315) construction
  line L480 (629.7295, 4.2315) -> (629.7295, 2.6714) construction
  line L481 (634.8662, 2.7666) -> (637.3394, 2.7666) construction
  line L482 (637.3394, 2.7666) -> (637.3394, 4.2124) construction
  line L483 (637.3394, 4.2124) -> (634.8662, 4.2124) construction
  line L484 (634.8662, 4.2124) -> (634.8662, 2.7666) construction
  line L485 (639.6414, 2.6714) -> (642.1717, 2.6714) construction
  line L486 (642.1717, 2.6714) -> (642.1717, 4.2885) construction
  line L487 (642.1717, 4.2885) -> (639.6414, 4.2885) construction
  line L488 (639.6414, 4.2885) -> (639.6414, 2.6714) construction
  line L489 (644.8542, 2.8046) -> (647.2894, 2.8046) construction
  line L490 (647.2894, 2.8046) -> (647.2894, 4.3456) construction
  line L491 (647.2894, 4.3456) -> (644.8542, 4.3456) construction
  line L492 (644.8542, 4.3456) -> (644.8542, 2.8046) construction
  line L493 (649.7436, 2.8046) -> (652.1598, 2.8046) construction
  line L494 (652.1598, 2.8046) -> (652.1598, 4.3456) construction
  line L495 (652.1598, 4.3456) -> (649.7436, 4.3456) construction
  line L496 (649.7436, 4.3456) -> (649.7436, 2.8046) construction
  line L497 (654.6901, 2.7095) -> (657.1823, 2.7095) construction
  line L498 (657.1823, 2.7095) -> (657.1823, 4.3456) construction
  line L499 (657.1823, 4.3456) -> (654.6901, 4.3456) construction
  line L500 (654.6901, 4.3456) -> (654.6901, 2.7095) construction
  line L501 (659.6365, 2.7856) -> (662.3, 2.7856) construction
  line L502 (662.3, 2.7856) -> (662.3, 4.2885) construction
  line L503 (662.3, 4.2885) -> (659.6365, 4.2885) construction
  line L504 (659.6365, 4.2885) -> (659.6365, 2.7856) construction
  line L505 (670.7233, 2.4938) -> (672.3503, 2.4938) construction
  line L506 (672.3503, 2.4938) -> (672.3503, 3.9241) construction
  line L507 (672.3503, 3.9241) -> (670.7233, 3.9241) construction
  line L508 (670.7233, 3.9241) -> (670.7233, 2.4938) construction
  line L509 (664.5, 2.8147) -> (667.4146, 2.8147) construction
  line L510 (667.4146, 2.8147) -> (667.4146, 4.5) construction
  line L511 (667.4146, 4.5) -> (664.5, 4.5) construction
  line L512 (664.5, 4.5) -> (664.5, 2.8147) construction
  arc A69 (599.5007, 5) -> (599.0007, 4.5) centre (599.5007, 4.5) ccw
  arc A70 (603.0007, 4.5) -> (602.5007, 5) centre (602.5007, 4.5) ccw
  arc A71 (602.5007, 2) -> (603.0007, 2.5) centre (602.5007, 2.5) ccw
  arc A72 (599.0007, 2.5) -> (599.5007, 2) centre (599.5007, 2.5) ccw
  arc A73 (604.5007, 5) -> (604.0007, 4.5) centre (604.5007, 4.5) ccw
  arc A74 (604.0007, 2.5) -> (604.5007, 2) centre (604.5007, 2.5) ccw
  arc A75 (607.5007, 2) -> (608.0007, 2.5) centre (607.5007, 2.5) ccw
  arc A76 (608.0007, 4.5) -> (607.5007, 5) centre (607.5007, 4.5) ccw
  arc A77 (609.5007, 5) -> (609.0007, 4.5) centre (609.5007, 4.5) ccw
  arc A78 (609.0007, 2.5) -> (609.5007, 2) centre (609.5007, 2.5) ccw
  arc A79 (613.0007, 4.5) -> (612.5007, 5) centre (612.5007, 4.5) ccw
  arc A80 (612.5007, 2) -> (613.0007, 2.5) centre (612.5007, 2.5) ccw
  arc A81 (614.5007, 5) -> (614.0007, 4.5) centre (614.5007, 4.5) ccw
  arc A82 (614.0007, 2.5) -> (614.5007, 2) centre (614.5007, 2.5) ccw
  arc A83 (617.5007, 2) -> (618.0007, 2.5) centre (617.5007, 2.5) ccw
  arc A84 (618.0007, 4.5) -> (617.5007, 5) centre (617.5007, 4.5) ccw
  arc A85 (619.0007, 2.5) -> (619.5007, 2) centre (619.5007, 2.5) ccw
  arc A86 (619.5007, 5) -> (619.0007, 4.5) centre (619.5007, 4.5) ccw
  arc A87 (623.0007, 4.5) -> (622.5007, 5) centre (622.5007, 4.5) ccw
  arc A88 (622.5007, 2) -> (623.0007, 2.5) centre (622.5007, 2.5) ccw
  arc A89 (624.0007, 2.5) -> (624.5007, 2) centre (624.5007, 2.5) ccw
  arc A90 (624.5007, 5) -> (624.0007, 4.5) centre (624.5007, 4.5) ccw
  arc A91 (628.0007, 4.5) -> (627.5007, 5) centre (627.5007, 4.5) ccw
  arc A92 (627.5007, 2) -> (628.0007, 2.5) centre (627.5007, 2.5) ccw
  arc A93 (629.0007, 2.5) -> (629.5007, 2) centre (629.5007, 2.5) ccw
  arc A94 (629.5007, 5) -> (629.0007, 4.5) centre (629.5007, 4.5) ccw
  arc A95 (633.0007, 4.5) -> (632.5007, 5) centre (632.5007, 4.5) ccw
  arc A96 (632.5007, 2) -> (633.0007, 2.5) centre (632.5007, 2.5) ccw
  arc A97 (634.0007, 2.5) -> (634.5007, 2) centre (634.5007, 2.5) ccw
  arc A98 (634.5007, 5) -> (634.0007, 4.5) centre (634.5007, 4.5) ccw
  arc A99 (638.0007, 4.5) -> (637.5007, 5) centre (637.5007, 4.5) ccw
  arc A100 (637.5007, 2) -> (638.0007, 2.5) centre (637.5007, 2.5) ccw
  arc A101 (639.0007, 2.5) -> (639.5007, 2) centre (639.5007, 2.5) ccw
  arc A102 (642.5007, 2) -> (643.0007, 2.5) centre (642.5007, 2.5) ccw
  arc A103 (643.0007, 4.5) -> (642.5007, 5) centre (642.5007, 4.5) ccw
  arc A104 (639.5007, 5) -> (639.0007, 4.5) centre (639.5007, 4.5) ccw
  arc A105 (644.0007, 2.5) -> (644.5007, 2) centre (644.5007, 2.5) ccw
  arc A106 (647.5007, 2) -> (648.0007, 2.5) centre (647.5007, 2.5) ccw
  arc A107 (648.0007, 4.5) -> (647.5007, 5) centre (647.5007, 4.5) ccw
  arc A108 (644.5007, 5) -> (644.0007, 4.5) centre (644.5007, 4.5) ccw
  arc A109 (649.0007, 2.5) -> (649.5007, 2) centre (649.5007, 2.5) ccw
  arc A110 (652.5007, 2) -> (653.0007, 2.5) centre (652.5007, 2.5) ccw
  arc A111 (653.0007, 4.5) -> (652.5007, 5) centre (652.5007, 4.5) ccw
  arc A112 (649.5007, 5) -> (649.0007, 4.5) centre (649.5007, 4.5) ccw
  arc A113 (654.5007, 5) -> (654.0007, 4.5) centre (654.5007, 4.5) ccw
  arc A114 (658.0007, 4.5) -> (657.5007, 5) centre (657.5007, 4.5) ccw
  arc A115 (657.5007, 2) -> (658.0007, 2.5) centre (657.5007, 2.5) ccw
  arc A116 (654.0007, 2.5) -> (654.5007, 2) centre (654.5007, 2.5) ccw
  arc A117 (659.0007, 2.5) -> (659.5007, 2) centre (659.5007, 2.5) ccw
  arc A118 (662.5007, 2) -> (663.0007, 2.5) centre (662.5007, 2.5) ccw
  arc A119 (663.0007, 4.5) -> (662.5007, 5) centre (662.5007, 4.5) ccw
  arc A120 (659.5007, 5) -> (659.0007, 4.5) centre (659.5007, 4.5) ccw
  arc A121 (664.5007, 5) -> (664.0007, 4.5) centre (664.5007, 4.5) ccw
  arc A122 (668.0007, 4.5) -> (667.5007, 5) centre (667.5007, 4.5) ccw
  arc A123 (667.5007, 2) -> (668.0007, 2.5) centre (667.5007, 2.5) ccw
  arc A124 (664.0007, 2.5) -> (664.5007, 2) centre (664.5007, 2.5) ccw
  arc A125 (669.0007, 2.5) -> (669.5007, 2) centre (669.5007, 2.5) ccw
  arc A126 (672.5007, 2) -> (673.0007, 2.5) centre (672.5007, 2.5) ccw
  arc A127 (673.0007, 4.5) -> (672.5007, 5) centre (672.5007, 4.5) ccw
  arc A128 (669.5007, 5) -> (669.0007, 4.5) centre (669.5007, 4.5) ccw
  arc A129 (674.5007, 5) -> (674.0007, 4.5) centre (674.5007, 4.5) ccw
  arc A130 (674.0007, 2.5) -> (674.5007, 2) centre (674.5007, 2.5) ccw
  arc A131 (677.5007, 2) -> (678.0007, 2.5) centre (677.5007, 2.5) ccw
  arc A132 (678.0007, 4.5) -> (677.5007, 5) centre (677.5007, 4.5) ccw
  arc A133 (679.5007, 5) -> (679.0007, 4.5) centre (679.5007, 4.5) ccw
  arc A134 (679.0007, 2.5) -> (679.5007, 2) centre (679.5007, 2.5) ccw
  arc A135 (682.5007, 2) -> (683.0007, 2.5) centre (682.5007, 2.5) ccw
  arc A136 (683.0007, 4.5) -> (682.5007, 5) centre (682.5007, 4.5) ccw
  arc A137 (684.5007, 5) -> (684.0007, 4.5) centre (684.5007, 4.5) ccw
  arc A138 (684.0007, 2.5) -> (684.5007, 2) centre (684.5007, 2.5) ccw
  arc A139 (688.0007, 4.5) -> (687.5007, 5) centre (687.5007, 4.5) ccw
  arc A140 (687.5007, 2) -> (688.0007, 2.5) centre (687.5007, 2.5) ccw
  arc A141 (688, 0.5) -> (687.5, 1) centre (687.5, 0.5) ccw
  arc A142 (687.5, -3) -> (688, -2.5) centre (687.5, -2.5) ccw
  arc A143 (684, -2.5) -> (684.5, -3) centre (684.5, -2.5) ccw
  arc A144 (684.5, 1) -> (684, 0.5) centre (684.5, 0.5) ccw
  arc A145 (682.5, -3) -> (683, -2.5) centre (682.5, -2.5) ccw
  arc A146 (679, -2.5) -> (679.5, -3) centre (679.5, -2.5) ccw
  arc A147 (679.5, 1) -> (679, 0.5) centre (679.5, 0.5) ccw
  arc A148 (683, 0.5) -> (682.5, 1) centre (682.5, 0.5) ccw
  arc A149 (677.5, -3) -> (678, -2.5) centre (677.5, -2.5) ccw
  arc A150 (674, -2.5) -> (674.5, -3) centre (674.5, -2.5) ccw
  arc A151 (674.5, 1) -> (674, 0.5) centre (674.5, 0.5) ccw
  arc A152 (678, 0.5) -> (677.5, 1) centre (677.5, 0.5) ccw
  arc A153 (672.5, -3) -> (673, -2.5) centre (672.5, -2.5) ccw
  arc A154 (669, -2.5) -> (669.5, -3) centre (669.5, -2.5) ccw
  arc A155 (673, 0.5) -> (672.5, 1) centre (672.5, 0.5) ccw
  arc A156 (669.5, 1) -> (669, 0.5) centre (669.5, 0.5) ccw
  arc A157 (667.5, -3) -> (668, -2.5) centre (667.5, -2.5) ccw
  arc A158 (661, -2.5) -> (661.5, -3) centre (661.5, -2.5) ccw
  arc A159 (661.5, 1) -> (661, 0.5) centre (661.5, 0.5) ccw
  arc A160 (668, 0.5) -> (667.5, 1) centre (667.5, 0.5) ccw
  arc A161 (688, -4.5) -> (687.5, -4) centre (687.5, -4.5) ccw
  arc A162 (684.5, -4) -> (684, -4.5) centre (684.5, -4.5) ccw
  arc A163 (684, -12.5) -> (684.5, -13) centre (684.5, -12.5) ccw
  arc A164 (687.5, -13) -> (688, -12.5) centre (687.5, -12.5) ccw
  arc A165 (683, -4.5) -> (682.5, -4) centre (682.5, -4.5) ccw
  arc A166 (682.5, -8) -> (683, -7.5) centre (682.5, -7.5) ccw
  arc A167 (679, -7.5) -> (679.5, -8) centre (679.5, -7.5) ccw
  arc A168 (679.5, -4) -> (679, -4.5) centre (679.5, -4.5) ccw
  arc A169 (678, -4.5) -> (677.5, -4) centre (677.5, -4.5) ccw
  arc A170 (677.5, -8) -> (678, -7.5) centre (677.5, -7.5) ccw
  arc A171 (674, -7.5) -> (674.5, -8) centre (674.5, -7.5) ccw
  arc A172 (674.5, -4) -> (674, -4.5) centre (674.5, -4.5) ccw
  arc A173 (678, -9.5) -> (677.5, -9) centre (677.5, -9.5) ccw
  arc A174 (677.5, -13) -> (678, -12.5) centre (677.5, -12.5) ccw
  arc A175 (679.5, -9) -> (679, -9.5) centre (679.5, -9.5) ccw
  arc A176 (683, -9.5) -> (682.5, -9) centre (682.5, -9.5) ccw
  arc A177 (679, -12.5) -> (679.5, -13) centre (679.5, -12.5) ccw
  arc A178 (684.5, -14) -> (684, -14.5) centre (684.5, -14.5) ccw
  arc A179 (688, -14.5) -> (687.5, -14) centre (687.5, -14.5) ccw
  arc A180 (687.5, -23) -> (688, -22.5) centre (687.5, -22.5) ccw
  arc A181 (684, -22.5) -> (684.5, -23) centre (684.5, -22.5) ccw
  arc A182 (682.5, -23) -> (683, -22.5) centre (682.5, -22.5) ccw
  arc A183 (683, -19.5) -> (682.5, -19) centre (682.5, -19.5) ccw
  arc A184 (679.5, -19) -> (679, -19.5) centre (679.5, -19.5) ccw
  arc A185 (679, -22.5) -> (679.5, -23) centre (679.5, -22.5) ccw
  arc A186 (682.5, -18) -> (683, -17.5) centre (682.5, -17.5) ccw
  arc A187 (683, -14.5) -> (682.5, -14) centre (682.5, -14.5) ccw
  arc A188 (679.5, -14) -> (679, -14.5) centre (679.5, -14.5) ccw
  arc A189 (679, -17.5) -> (679.5, -18) centre (679.5, -17.5) ccw
  arc A190 (677.5, -18) -> (678, -17.5) centre (677.5, -17.5) ccw
  arc A191 (678, -14.5) -> (677.5, -14) centre (677.5, -14.5) ccw
  arc A192 (674.5, -14) -> (674, -14.5) centre (674.5, -14.5) ccw
  arc A193 (674, -17.5) -> (674.5, -18) centre (674.5, -17.5) ccw
  arc A194 (678, -19.5) -> (677.5, -19) centre (677.5, -19.5) ccw
  arc A195 (677.5, -23) -> (678, -22.5) centre (677.5, -22.5) ccw
  arc A196 (669, -22.5) -> (669.5, -23) centre (669.5, -22.5) ccw
  arc A197 (669.5, -19) -> (669, -19.5) centre (669.5, -19.5) ccw
  arc A198 (672.5, -18) -> (673, -17.5) centre (672.5, -17.5) ccw
  arc A199 (673, -14.5) -> (672.5, -14) centre (672.5, -14.5) ccw
  arc A200 (669.5, -14) -> (669, -14.5) centre (669.5, -14.5) ccw
  arc A201 (669, -17.5) -> (669.5, -18) centre (669.5, -17.5) ccw
  arc A202 (674, -12.5) -> (674.5, -13) centre (674.5, -12.5) ccw
  arc A203 (674.5, -9) -> (674, -9.5) centre (674.5, -9.5) ccw
  arc A204 (673, -9.5) -> (672.5, -9) centre (672.5, -9.5) ccw
  arc A205 (672.5, -13) -> (673, -12.5) centre (672.5, -12.5) ccw
  arc A206 (669, -12.5) -> (669.5, -13) centre (669.5, -12.5) ccw
  arc A207 (669.5, -9) -> (669, -9.5) centre (669.5, -9.5) ccw
  arc A208 (672.5, -8) -> (673, -7.5) centre (672.5, -7.5) ccw
  arc A209 (673, -4.5) -> (672.5, -4) centre (672.5, -4.5) ccw
  arc A210 (669.5, -4) -> (669, -4.5) centre (669.5, -4.5) ccw
  arc A211 (669, -7.5) -> (669.5, -8) centre (669.5, -7.5) ccw
  arc A212 (667.5, -23) -> (668, -22.5) centre (667.5, -22.5) ccw
  arc A213 (668, -19.5) -> (667.5, -19) centre (667.5, -19.5) ccw
  arc A214 (664.5, -19) -> (664, -19.5) centre (664.5, -19.5) ccw
  arc A215 (664, -22.5) -> (664.5, -23) centre (664.5, -22.5) ccw
  arc A216 (662.5, -23) -> (663, -22.5) centre (662.5, -22.5) ccw
  arc A217 (663, -21.6515) -> (662.5, -21.1515) centre (662.5, -21.6515) ccw
  arc A218 (659.5138, -21.1515) -> (659.0138, -21.6515) centre (659.5138, -21.6515) ccw
  arc A219 (659.0138, -22.5) -> (659.5138, -23) centre (659.5138, -22.5) ccw
  arc A220 (662.5, -20.702) -> (663, -20.202) centre (662.5, -20.202) ccw
  arc A221 (663, -19.5) -> (662.5, -19) centre (662.5, -19.5) ccw
  arc A222 (659.5138, -19) -> (659.0138, -19.5) centre (659.5138, -19.5) ccw
  arc A223 (659.0138, -20.202) -> (659.5138, -20.702) centre (659.5138, -20.202) ccw
  arc A224 (667.5, -18) -> (668, -17.5) centre (667.5, -17.5) ccw
  arc A225 (668, -14.5) -> (667.5, -14) centre (667.5, -14.5) ccw
  arc A226 (660.5, -14) -> (660, -14.5) centre (660.5, -14.5) ccw
  arc A227 (660, -17.5) -> (660.5, -18) centre (660.5, -17.5) ccw
  arc A228 (667.5, -13) -> (668, -12.5) centre (667.5, -12.5) ccw
  arc A229 (668, -9.5) -> (667.5, -9) centre (667.5, -9.5) ccw
  arc A230 (661.5, -9) -> (661, -9.5) centre (661.5, -9.5) ccw
  arc A231 (661, -12.5) -> (661.5, -13) centre (661.5, -12.5) ccw
  arc A232 (667.5, -8) -> (668, -7.5) centre (667.5, -7.5) ccw
  arc A233 (668, -4.5) -> (667.5, -4) centre (667.5, -4.5) ccw
  arc A234 (664.5, -4) -> (664, -4.5) centre (664.5, -4.5) ccw
  arc A235 (664, -7.5) -> (664.5, -8) centre (664.5, -7.5) ccw
  arc A236 (662.5, -8) -> (663, -7.5) centre (662.5, -7.5) ccw
  arc A237 (663, -4.5) -> (662.5, -4) centre (662.5, -4.5) ccw
  arc A238 (659.5, -4) -> (659, -4.5) centre (659.5, -4.5) ccw
  arc A239 (659, -7.5) -> (659.5, -8) centre (659.5, -7.5) ccw
  arc A240 (660, -9.5) -> (659.5, -9) centre (659.5, -9.5) ccw
  arc A241 (656.5, -9) -> (656, -9.5) centre (656.5, -9.5) ccw
  arc A242 (656, -12.5) -> (656.5, -13) centre (656.5, -12.5) ccw
  arc A243 (659.5, -13) -> (660, -12.5) centre (659.5, -12.5) ccw
  arc A244 (659, -14.5) -> (658.5, -14) centre (658.5, -14.5) ccw
  arc A245 (655.5, -14) -> (655, -14.5) centre (655.5, -14.5) ccw
  arc A246 (655, -17.5) -> (655.5, -18) centre (655.5, -17.5) ccw
  arc A247 (658.5, -18) -> (659, -17.5) centre (658.5, -17.5) ccw
  arc A248 (658, -19.5) -> (657.5, -19) centre (657.5, -19.5) ccw
  arc A249 (654.5, -19) -> (654, -19.5) centre (654.5, -19.5) ccw
  arc A250 (654, -22.5) -> (654.5, -23) centre (654.5, -22.5) ccw
  arc A251 (657.5, -23) -> (658, -22.5) centre (657.5, -22.5) ccw
  arc A252 (652.5, -23) -> (653, -22.5) centre (652.5, -22.5) ccw
  arc A253 (653, -19.5) -> (652.5, -19) centre (652.5, -19.5) ccw
  arc A254 (649.5, -19) -> (649, -19.5) centre (649.5, -19.5) ccw
  arc A255 (649, -22.5) -> (649.5, -23) centre (649.5, -22.5) ccw
  arc A256 (647.5, -23) -> (648, -22.5) centre (647.5, -22.5) ccw
  arc A257 (644, -22.5) -> (644.5, -23) centre (644.5, -22.5) ccw
  arc A258 (644.5, -19) -> (644, -19.5) centre (644.5, -19.5) ccw
  arc A259 (648, -19.5) -> (647.5, -19) centre (647.5, -19.5) ccw
  arc A260 (653.5, -18) -> (654, -17.5) centre (653.5, -17.5) ccw
  arc A261 (654, -14.5) -> (653.5, -14) centre (653.5, -14.5) ccw
  arc A262 (650.5, -14) -> (650, -14.5) centre (650.5, -14.5) ccw
  arc A263 (650, -17.5) -> (650.5, -18) centre (650.5, -17.5) ccw
  arc A264 (648.5, -18) -> (649, -17.5) centre (648.5, -17.5) ccw
  arc A265 (649, -14.5) -> (648.5, -14) centre (648.5, -14.5) ccw
  arc A266 (645.5, -14) -> (645, -14.5) centre (645.5, -14.5) ccw
  arc A267 (645, -17.5) -> (645.5, -18) centre (645.5, -17.5) ccw
  arc A268 (643.5, -18) -> (644, -17.5) centre (643.5, -17.5) ccw
  arc A269 (644, -14.5) -> (643.5, -14) centre (643.5, -14.5) ccw
  arc A270 (640.5, -14) -> (640, -14.5) centre (640.5, -14.5) ccw
  arc A271 (640, -17.5) -> (640.5, -18) centre (640.5, -17.5) ccw
  arc A272 (643, -19.5) -> (642.5, -19) centre (642.5, -19.5) ccw
  arc A273 (642.5, -23) -> (643, -22.5) centre (642.5, -22.5) ccw
  arc A274 (638.5, -18) -> (639, -17.5) centre (638.5, -17.5) ccw
  arc A275 (635, -17.5) -> (635.5, -18) centre (635.5, -17.5) ccw
  arc A276 (635.5, -14) -> (635, -14.5) centre (635.5, -14.5) ccw
  arc A277 (639, -14.5) -> (638.5, -14) centre (638.5, -14.5) ccw
  arc A278 (654.5, -13) -> (655, -12.5) centre (654.5, -12.5) ccw
  arc A279 (651, -12.5) -> (651.5, -13) centre (651.5, -12.5) ccw
  arc A280 (649.5, -13) -> (650, -12.5) centre (649.5, -12.5) ccw
  arc A281 (646, -12.5) -> (646.5, -13) centre (646.5, -12.5) ccw
  arc A282 (644.5, -13) -> (645, -12.5) centre (644.5, -12.5) ccw
  arc A283 (641, -12.5) -> (641.5, -13) centre (641.5, -12.5) ccw
  arc A284 (639.5, -13) -> (640, -12.5) centre (639.5, -12.5) ccw
  arc A285 (636, -12.5) -> (636.5, -13) centre (636.5, -12.5) ccw
  arc A286 (634.5, -13) -> (635, -12.5) centre (634.5, -12.5) ccw
  arc A287 (631, -12.5) -> (631.5, -13) centre (631.5, -12.5) ccw
  arc A288 (633.5, -18) -> (634, -17.5) centre (633.5, -17.5) ccw
  arc A289 (630, -17.5) -> (630.5, -18) centre (630.5, -17.5) ccw
  arc A290 (634, -14.5) -> (633.5, -14) centre (633.5, -14.5) ccw
  arc A291 (628.5, -18) -> (629, -17.5) centre (628.5, -17.5) ccw
  arc A292 (655, -9.5) -> (654.5, -9) centre (654.5, -9.5) ccw
  arc A293 (651.5, -9) -> (651, -9.5) centre (651.5, -9.5) ccw
  arc A294 (650, -9.5) -> (649.5, -9) centre (649.5, -9.5) ccw
  arc A295 (646.5, -9) -> (646, -9.5) centre (646.5, -9.5) ccw
  arc A296 (645, -9.5) -> (644.5, -9) centre (644.5, -9.5) ccw
  arc A297 (641.5, -9) -> (641, -9.5) centre (641.5, -9.5) ccw
  arc A298 (640, -9.5) -> (639.5, -9) centre (639.5, -9.5) ccw
  arc A299 (636.5, -9) -> (636, -9.5) centre (636.5, -9.5) ccw
  arc A300 (635, -9.5) -> (634.5, -9) centre (634.5, -9.5) ccw
  arc A301 (631.5, -9) -> (631, -9.5) centre (631.5, -9.5) ccw
  arc A302 (630, -9.5) -> (629.5, -9) centre (629.5, -9.5) ccw
  arc A303 (626.5, -9) -> (626, -9.5) centre (626.5, -9.5) ccw
  arc A304 (597.5, 1) -> (597, 0.5) centre (597.5, 0.5) ccw
  arc A305 (600, 0.5) -> (599.5, 1) centre (599.5, 0.5) ccw
  arc A306 (597, -2.5) -> (597.5, -3) centre (597.5, -2.5) ccw
  arc A307 (599.5, -3) -> (600, -2.5) centre (599.5, -2.5) ccw